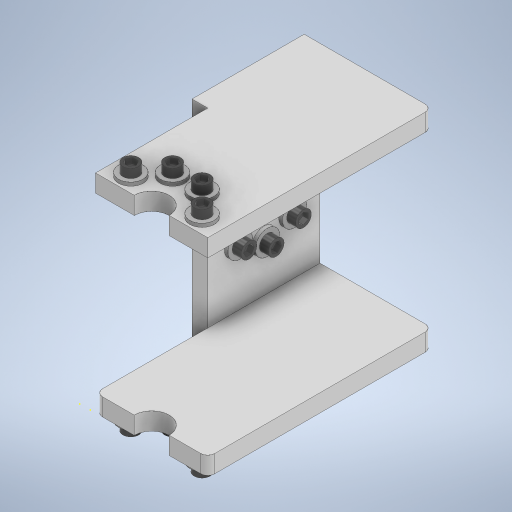
# Autodesk Inventor part: link_manip
Saved by Autodesk Inventor 2024 (Build 280153000, 153)
## iProperties
Created: 2024-10-14
Part Number: link_manip
Material: Genérico
Document SubType Name: Modeling
Designer: robof
Density: 1 g/cm^3
Appearance: Padrão
Author: robof
Autodesk Inventor part; units mm, degrees
ref_plane "YZ Plane" through (0, 0, 0) normal (1, 0, 0) x (0, 1, 0)
ref_plane "XZ Plane" through (0, 0, 0) normal (0, 1, 0) x (-1, 0, 0)
ref_plane "XY Plane" through (0, 0, 0) normal (0, 0, 1) x (1, 0, 0)
sketch "Esboço1" plane through (0, 0, 0) normal (0, 1, 0) x (-1, 0, 0)
  line L0 (0, 0) -> (-32, 0)
  line L1 (-32, 0) -> (-32, -64)
  line L2 (-32, -64) -> (0, -64)
  line L3 (0, -64) -> (0, 0)
  dimension "d0" = 32
  dimension "d1" = 64
  constraints: 8 end point, 2 parallel, 1 horizontal, 1 perpendicular
  measures "d0" distance of L2.end L1.end
  measures "d1" distance of L1.end L0.end
extrude "Extrusão1" add sketch "Esboço1" along normal blind 5
sketch "Esboço2" plane through (0, 5, 0) normal (0, 1, 0) x (1, 0, 0)
  line L0 (32, 64) -> (0, 64) projected
  line L1 (0, 64) -> (-4.5, 64)
  line L2 (-4.5, 64) -> (-4.5, 35.5)
  line L3 (-4.5, 35.5) -> (0, 35.5)
  line L4 (0, 35.5) -> (0, 64)
  point P0 (0, 0)
  dimension "d4" = 4.5
  dimension "d5" = 28.5
  constraints: 8 end point, 2 parallel, 1 horizontal, 1 perpendicular
  measures "d4" distance of L3.end L2.end
  measures "d5" distance of L2.end L1.end
extrude "Extrusão2" add sketch "Esboço2" along normal blind 59.3
sketch "Esboço3" plane through (0, 5, 0) normal (0, -1, 0) x (1, 0, 0)
  line L0 (0, -64) -> (-4.5, -64) projected
  line L1 (0, -64) -> (0, -35.5) projected
  line L2 (-4.5, -64) -> (0, -64)
  line L3 (0, -64) -> (0, -35.5)
  line L4 (0, -35.5) -> (-4.5, -35.5)
  line L5 (-4.5, -35.5) -> (-4.5, -64)
  point P0 (0, 0)
  constraints: 8 end point, 2 parallel, 1 horizontal, 1 perpendicular
extrude "Extrusão3" add sketch "Esboço3" along normal blind 5
sketch "Esboço4" plane through (0, 64.3, 0) normal (0, 1, 0) x (1, 0, 0)
  line L0 (-4.5, 35.5) -> (-4.5, 64) projected
  line L1 (0, 35.5) -> (0, 64) projected
  line L2 (-4.5, 64) -> (0, 64)
  line L3 (0, 64) -> (0, 35.5)
  line L4 (0, 35.5) -> (-4.5, 35.5)
  line L5 (-4.5, 35.5) -> (-4.5, 64)
  point P0 (0, 0)
  constraints: 8 end point, 2 parallel, 1 horizontal, 1 perpendicular
extrude "Extrusão4" cut sketch "Esboço4" against normal blind 5
sketch "Esboço5" plane through (0, 59.3, 0) normal (0, 1, 0) x (1, 0, 0)
  line L0 (0, 64) -> (0, 35.5) projected
  line L1 (0, 0) -> (32, 0) projected
  line L2 (0, 64) -> (32, 64)
  line L3 (32, 64) -> (32, 0)
  line L4 (32, 0) -> (0, 0)
  line L5 (0, 0) -> (0, 64)
  constraints: 8 end point, 2 parallel, 1 horizontal, 1 perpendicular
extrude "Extrusão5" add sketch "Esboço5" against normal blind 5
sketch "Esboço6" plane through (0, 59.3, 0) normal (0, 1, 0) x (1, 0, 0)
  line L0 (0, 0) -> (32, 0) projected
  circle A0 centre (16, 0) radius 4.975
  point P0 (20.975, 0)
  point P1 (11.025, 0)
  dimension "d14" = 9.95
  constraints: 1 centre point, 1 midpoint
  measures "d14" diameter of A0
extrude "Extrusão6" cut sketch "Esboço6" against normal blind 100 contours A0 L0 picked at (17.4684, 0.7707)
sketch "Esboço7" plane through (0, 0, 0) normal (0, -1, 0) x (1, 0, 0)
  arc A0 (11.025, 0) -> (20.975, 0) centre (16, 0) ccw projected
  line L0 (16, 0) -> (16, -11.7992)
  line L1 (16, 0) -> (24.7548, -8.7548)
  line L2 (16, 0) -> (28.3812, 0) construction
  line L3 (16, 0) -> (21.1285, -12.3812)
  line L4 (16, 0) -> (29.4013, 0) construction
  line L5 (16, 0) -> (27.5056, -4.7658)
  line L6 (16, 0) -> (28.4535, 0) construction
  arc A1 (11.025, 0) -> (20.975, 0) centre (16, 0) ccw
  line L7 (16, 0) -> (7.2452, -8.7548)
  line L8 (16, 0) -> (10.8715, -12.3812)
  line L9 (16, 0) -> (4.4944, -4.7658)
  line L10 (16, 0) -> (26.1627, -4.2095)
  circle A2 centre (26.1627, -4.2095) radius 3.5
  circle A3 centre (20.2095, -10.1627) radius 3.5
  circle A4 centre (5.8373, -4.2095) radius 3.5
  circle A5 centre (11.7905, -10.1627) radius 3.5
  point P0 (0, 0)
  dimension "d17" = 45
  dimension "d18" = 67.5
  dimension "d19" = 22.5
  dimension "d20" = 11
  dimension "d21" = 7
  constraints: 22 end point, 8 symmetric about line, 5 centre point, 3 equal length, 3 horizontal, 2 point on circle, 1 coincident, 1 point on line, 1 vertical, 4 other
  measures "d17" angle of L1 L2
  measures "d18" angle of L3 L4
  measures "d19" angle of L5 L6
  measures "d20" distance of L0.start L10.end
  measures "d21" diameter of A2
extrude "Extrusão7" add sketch "Esboço7" along normal blind 1 contours A2 | A3 | A5 | A4
sketch "Esboço8" plane through (5.8373, -1, -4.2095) normal (0, -1, 0) x (1, 0, 0)
  circle A0 centre (0, 0) radius 2.25
  circle A1 centre (5.9532, -5.9532) radius 3.5 projected
  circle A2 centre (5.9532, -5.9532) radius 2.25
  circle A3 centre (14.3722, -5.9532) radius 3.5 projected
  circle A4 centre (14.3722, -5.9532) radius 2.25
  circle A5 centre (20.3253, 0) radius 3.5 projected
  circle A6 centre (20.3253, 0) radius 2.25
  point P0 (-5.8373, 4.2095)
  dimension "d24" = 4.5
  dimension "d25" = 4.5
  dimension "d26" = 4.5
  dimension "d27" = 4.5
  constraints: 4 centre point, 3 coincident
  measures "d24" diameter of A0
  measures "d25" diameter of A2
  measures "d26" diameter of A4
  measures "d27" diameter of A6
extrude "Extrusão8" add sketch "Esboço8" along normal blind 2.5 contours A0 | A2 | A4 | A6
sketch "Esboço9" plane through (5.8373, -3.5, -4.2095) normal (0, -1, 0) x (1, 0, 0)
  line L0 (-1.5951, 0) -> (-0.7976, 1.3814)
  line L1 (-0.7976, 1.3814) -> (0.7976, 1.3814)
  line L2 (0.7976, 1.3814) -> (1.5951, 0)
  line L3 (1.5951, 0) -> (0.7976, -1.3814)
  line L4 (0.7976, -1.3814) -> (-0.7976, -1.3814)
  line L5 (-0.7976, -1.3814) -> (-1.5951, 0)
  arc A0 (5.1877, 4.2095) -> (15.1377, 4.2095) centre (10.1627, 4.2095) ccw projected
  line L6 (10.1627, 4.2095) -> (-1.1963, -7.1495)
  line L7 (10.1627, 4.2095) -> (26.2267, 4.2095) construction
  line L8 (10.1627, 4.2095) -> (19.9498, -5.5776)
  line L9 (10.1627, 4.2095) -> (10.1627, -8.2153)
  line L10 (5.9532, -7.5483) -> (7.3346, -6.7507)
  line L11 (7.3346, -6.7507) -> (7.3346, -5.1556)
  line L12 (7.3346, -5.1556) -> (5.9532, -4.3581)
  line L13 (5.9532, -4.3581) -> (4.5718, -5.1556)
  line L14 (4.5718, -5.1556) -> (4.5718, -6.7507)
  line L15 (4.5718, -6.7507) -> (5.9532, -7.5483)
  line L16 (21.9205, 0) -> (21.1229, 1.3814)
  line L17 (21.1229, 1.3814) -> (19.5278, 1.3814)
  line L18 (19.5278, 1.3814) -> (18.7302, 0)
  line L19 (18.7302, 0) -> (19.5278, -1.3814)
  line L20 (19.5278, -1.3814) -> (21.1229, -1.3814)
  line L21 (21.1229, -1.3814) -> (21.9205, 0)
  line L22 (14.3722, -7.5483) -> (12.9908, -6.7507)
  line L23 (12.9908, -6.7507) -> (12.9908, -5.1556)
  line L24 (12.9908, -5.1556) -> (14.3722, -4.3581)
  line L25 (14.3722, -4.3581) -> (15.7536, -5.1556)
  line L26 (15.7536, -5.1556) -> (15.7536, -6.7507)
  line L27 (15.7536, -6.7507) -> (14.3722, -7.5483)
  point P0 (-5.8373, 4.2095)
  point P1 (0, 0)
  point P2 (5.9532, -5.9532)
  point P3 (20.3253, 0)
  point P4 (21.5217, -7.1495)
  point P5 (14.3722, -5.9532)
  dimension "d30" = 135
  constraints: 56 end point, 22 symmetric about line, 1 equal length, 1 horizontal, 1 vertical, 13 other
  measures "d30" angle of L6 L7
extrude "Extrusão9" cut sketch "Esboço9" against normal blind 1.5 contours L0 L1 L2 L3 L4 L5 | L15 L14 L13 L12 L11 L10 | L21 L20 L19 L18 L17 L16 | L22 L23 L24 L25 L26 L27
sketch "Esboço10" plane through (0, 59.3, 0) normal (0, 1, 0) x (1, 0, 0)
  circle A0 centre (20.2095, 10.1627) radius 3.5 projected
  circle A1 centre (20.2095, 10.1627) radius 3.5
  circle A2 centre (26.1627, 4.2095) radius 2.25 projected
  circle A3 centre (26.1627, 4.2095) radius 3.5
  circle A4 centre (11.7905, 10.1627) radius 2.25 projected
  circle A5 centre (11.7905, 10.1627) radius 3.5
  circle A6 centre (5.8373, 4.2095) radius 3.5
  point P0 (0, 0)
  constraints: 4 centre point, 3 coincident
extrude "Extrusão10" add sketch "Esboço10" along normal blind 1 contours A0 | A2 | A3 | A4 | A5 | A6
sketch "Esboço11" plane through (5.8373, 60.3, -4.2095) normal (0, 1, 0) x (1, 0, 0)
  circle A0 centre (0, 0) radius 2.25
  circle A1 centre (5.9532, 5.9532) radius 2.25 projected
  circle A2 centre (5.9532, 5.9532) radius 2.25
  circle A3 centre (14.3722, 5.9532) radius 3.5 projected
  circle A4 centre (14.3722, 5.9532) radius 2.25
  circle A5 centre (20.3253, 0) radius 3.5 projected
  circle A6 centre (20.3253, 0) radius 2.25
  point P0 (-5.8373, -4.2095)
  constraints: 4 centre point, 3 coincident
extrude "Extrusão11" add sketch "Esboço11" along normal blind 2.5 contours A0 | A1 | A4 | A6
sketch "Esboço12" plane through (5.8373, 62.8, -4.2095) normal (0, 1, 0) x (1, 0, 0)
  circle A0 centre (0, 0) radius 2.25 projected
  line L0 (0.7976, 1.3814) -> (-0.7976, 1.3814) projected
  line L1 (0.7976, 1.3814) -> (1.5951, 0)
  line L2 (1.5951, 0) -> (0.7976, -1.3814)
  line L3 (0.7976, -1.3814) -> (-0.7976, -1.3814)
  line L4 (-0.7976, -1.3814) -> (-1.5951, 0)
  line L5 (-1.5951, 0) -> (-0.7976, 1.3814)
  line L6 (-0.7976, 1.3814) -> (0.7976, 1.3814)
  circle A1 centre (5.9532, 5.9532) radius 2.25 projected
  line L7 (7.3346, 6.7507) -> (5.9532, 7.5483) projected
  line L8 (5.9532, 7.5483) -> (7.3346, 6.7507)
  line L9 (7.3346, 6.7507) -> (7.3346, 5.1556)
  line L10 (7.3346, 5.1556) -> (5.9532, 4.3581)
  line L11 (5.9532, 4.3581) -> (4.5718, 5.1556)
  line L12 (4.5718, 5.1556) -> (4.5718, 6.7507)
  line L13 (4.5718, 6.7507) -> (5.9532, 7.5483)
  circle A2 centre (14.3722, 5.9532) radius 2.25 projected
  line L14 (12.9908, 5.1556) -> (14.3722, 4.3581) projected
  line L15 (12.9908, 5.1556) -> (12.9908, 6.7507)
  line L16 (12.9908, 6.7507) -> (14.3722, 7.5483)
  line L17 (14.3722, 7.5483) -> (15.7536, 6.7507)
  line L18 (15.7536, 6.7507) -> (15.7536, 5.1556)
  line L19 (15.7536, 5.1556) -> (14.3722, 4.3581)
  line L20 (14.3722, 4.3581) -> (12.9908, 5.1556)
  circle A3 centre (20.3253, 0) radius 2.25 projected
  line L21 (19.5277, -1.3814) -> (18.7302, 0.0001)
  line L22 (18.7302, 0.0001) -> (19.5278, 1.3815)
  line L23 (19.5278, 1.3815) -> (21.123, 1.3814)
  line L24 (21.123, 1.3814) -> (21.9205, -0.0001)
  line L25 (21.9205, -0.0001) -> (21.1229, -1.3815)
  line L26 (21.1229, -1.3815) -> (19.5277, -1.3814)
  point P0 (-5.8373, -4.2095)
  constraints: 48 end point, 4 coincident, 1 point on line, 52 other
extrude "Extrusão12" cut sketch "Esboço12" against normal blind 1.5 contours L1 L2 L3 L4 L5 L0 | L9 L10 L11 L12 L13 L7 | L15 L16 L17 L18 L19 L14 | L21 L22 L23 L24 L25 L26
fillet "Arredondamento1" radius 2 6 edges at (0, 2.5, 0) (32, 2.5, 0) (32, 2.5, -64) (32, 56.8, -64) (0, 56.8, -35.5) (0, 2.5, -35.5)
sketch "Esboço13" plane through (0, 5, -35.5) normal (1, 0, 0) x (0, 0, -1)
  line L0 (0, 0) -> (0, 49.3) projected
  line L1 (0, 24.65) -> (28.5, 24.65)
  line L2 (28.5, 0) -> (28.5, 49.3) projected
  circle A0 centre (14.25, 24.65) radius 5.85
  point P0 (-35.5, -5)
  dimension "d40" = 11.7
  constraints: 3 midpoint, 2 end point, 1 centre point
  measures "d40" diameter of A0
extrude "Extrusão13" cut sketch "Esboço13" against normal blind 1.5
sketch "Esboço14" plane through (-1.5, 29.65, -49.75) normal (1, 0, 0) x (0, 0, -1)
  point P0 (-49.75, -29.65)
sketch "Esboço15" plane through (0, 5, -35.5) normal (1, 0, 0) x (0, 0, -1)
  circle A0 centre (14.25, 24.65) radius 5.85 projected
  circle A1 centre (14.25, 24.65) radius 5.85
  point P0 (-35.5, -5)
  constraints: 1 centre point, 1 coincident
extrude "Extrusão14" add sketch "Esboço15" against normal blind 10
sketch "Esboço16" plane through (0, 5, -35.5) normal (1, 0, 0) x (0, 0, -1)
  line L0 (0, 0) -> (0, 49.3) projected
  line L1 (0, 24.65) -> (28.5, 24.65)
  line L2 (28.5, 0) -> (28.5, 49.3) projected
  circle A0 centre (14.25, 24.65) radius 5.85
  point P0 (-35.5, -5)
  constraints: 3 midpoint, 2 end point, 1 centre point
extrude "Extrusão15" cut sketch "Esboço16" against normal blind 10
sketch "Esboço17" plane through (0, 5, -35.5) normal (1, 0, 0) x (0, 0, -1)
  line L0 (14.25, 24.65) -> (28.5632, 24.65) construction
  line L1 (0, 0) -> (0, 49.3) projected
  line L2 (0, 24.65) -> (28.5632, 24.65)
  circle A0 centre (14.25, 24.65) radius 5.85 projected
  circle A1 centre (14.25, 24.65) radius 5.85
  point P0 (-35.5, -5)
  constraints: 4 end point, 1 centre point, 1 coincident, 1 collinear, 1 horizontal, 1 midpoint
extrude "Extrusão16" add sketch "Esboço17" against normal blind 5
sketch "Esboço18" plane through (-4.5, 0, -35.5) normal (0, 0, 1) x (1, 0, 0)
  line L0 (0, 59.3) -> (4.5, 59.3)
  line L1 (4.5, 59.3) -> (4.5, 0)
  line L2 (4.5, 0) -> (0, 0)
  line L3 (0, 0) -> (0, 59.3)
  constraints: 8 end point, 2 parallel, 1 horizontal, 1 perpendicular
extrude "Extrusão17" add sketch "Esboço18" along normal blind 3.5
sketch "Esboço19" plane through (-5, 29.65, -49.75) normal (-1, 0, 0) x (0, 0, 1)
  circle A0 centre (0, 0) radius 5.85 projected
  circle A1 centre (0, 0) radius 5.85
  point P0 (49.75, -29.65)
  constraints: 1 centre point, 1 coincident
extrude "Extrusão18" cut sketch "Esboço19" against normal blind 0.5
sketch "Esboço20" plane through (0, 5, -64) normal (1, 0, 0) x (0, 0, -1)
  line L0 (-32, 54.3) -> (-32, -5) projected
  line L1 (-32, 24.65) -> (0, 24.65)
  line L2 (0, -5) -> (0, 54.3) projected
  circle A0 centre (-16, 24.65) radius 5.9
  line L3 (-16, 24.65) -> (-8.2218, 16.8718)
  line L4 (-16, 24.65) -> (-5, 24.65) construction
  line L5 (-16, 24.65) -> (-16, 13.65)
  line L6 (-16, 24.65) -> (-8.2218, 32.4282)
  line L7 (-16, 24.65) -> (-16, 35.65)
  line L8 (-16, 24.65) -> (-23.7782, 16.8718)
  line L9 (-16, 24.65) -> (-23.7782, 32.4282)
  circle A1 centre (-8.2218, 32.4282) radius 3.5
  circle A2 centre (-16, 35.65) radius 3.5
  circle A3 centre (-23.7782, 32.4282) radius 3.5
  circle A4 centre (-23.7782, 16.8718) radius 3.5
  circle A5 centre (-16, 13.65) radius 3.5
  circle A6 centre (-8.2218, 16.8718) radius 3.5
  line L10 (-16, 24.65) -> (-5, 24.65)
  circle A7 centre (-5, 24.65) radius 3.5
  line L11 (-16, 24.65) -> (-27, 24.65)
  circle A8 centre (-27, 24.65) radius 3.5
  point P0 (-64, -5)
  point P1 (-30.5, 24.65)
  point P2 (-23.5, 24.65)
  dimension "d60" = 11.8
  dimension "d61" = 11
  dimension "d62" = 45
  dimension "d63" = 11
  dimension "d64" = 7
  dimension "d65" = 7
  dimension "d66" = 7
  dimension "d67" = 7
  dimension "d68" = 7
  dimension "d69" = 7
  dimension "d70" = 11
  dimension "d71" = 7
  dimension "d72" = 11
  dimension "d73" = 7
  constraints: 20 end point, 9 centre point, 8 coincident, 4 symmetric about line, 3 midpoint, 1 collinear, 1 equal length, 1 horizontal, 1 point on line, 1 vertical
  measures "d60" diameter of A0
  measures "d61" distance of L3.start L3.end
  measures "d62" angle of L3 L4
  measures "d63" distance of L3.start L5.end
  measures "d64" diameter of A1
  measures "d65" diameter of A2
  measures "d66" diameter of A3
  measures "d67" diameter of A4
  measures "d68" diameter of A5
  measures "d69" diameter of A6
  measures "d70" distance of L3.start L4.end
  measures "d71" diameter of A7
  measures "d72" distance of L3.start L11.end
  measures "d73" diameter of A8
extrude "Extrusão19" add sketch "Esboço20" along normal blind 1 contours L1 A8 | A3 | A2 | A1 | A7 L1 | L1 A7 | A6 | A5 | A4 | A0 L9 L1 | L1 L8 A0 | L6 A0 L1 | L1 A0 L3 | L3 A0 L5 | L7 A0 L6 | L9 A0 L7 | L5 A0 L8 picked at (-24.7006, 24.3708)
sketch "Esboço21" plane through (0, 5, -64) normal (1, 0, 0) x (0, 0, -1)
  line L0 (-23.5, 24.65) -> (-30.5, 24.65) projected
  circle A0 centre (-27, 24.65) radius 3.5
  point P0 (-64, -5)
  constraints: 1 midpoint, 3 other
extrude "Extrusão20" add sketch "Esboço21" along normal blind 1 contours L0 A0 picked at (-26.1267, 25.4236)
sketch "Esboço22" plane through (1, 29.65, -48) normal (1, 0, 0) x (0, 0, -1)
  circle A0 centre (0, 0) radius 5.9 projected
  circle A1 centre (0, 0) radius 5.9
  point P0 (-48, -29.65)
  constraints: 1 centre point, 1 coincident
extrude "Extrusão21" cut sketch "Esboço22" against normal blind 3
sketch "Esboço23" plane through (-2, 29.65, -48) normal (1, 0, 0) x (0, 0, -1)
  circle A0 centre (0, 0) radius 5.9 projected
  circle A1 centre (0, 0) radius 5.9
  point P0 (-48, -29.65)
  constraints: 1 centre point, 1 coincident
extrude "Extrusão22" cut sketch "Esboço23" against normal blind 20
sketch "Esboço24" plane through (1, 29.65, -59) normal (1, 0, 0) x (0, 0, -1)
  circle A0 centre (0, 0) radius 3.5 projected
  circle A1 centre (0, 0) radius 2.25
  circle A2 centre (-11, 0) radius 5.9 projected
  line L0 (-11, 0) -> (2.7014, 0) construction
  circle A3 centre (-11, -11) radius 2.25
  line L1 (-11, 0) -> (4.8079, 0)
  circle A4 centre (-11, -11) radius 2.25
  circle A5 centre (0, 0) radius 2.25
  circle A6 centre (-22, 0) radius 2.25
  circle A7 centre (-11, 11) radius 3.5 projected
  circle A8 centre (-11, 11) radius 2.25
  circle A9 centre (-3.2218, 7.7782) radius 2.25
  circle A10 centre (-11, 11) radius 2.25
  circle A11 centre (-18.7782, 7.7782) radius 2.25
  circle A12 centre (-22, 0) radius 2.25
  circle A13 centre (-18.7782, -7.7782) radius 2.25
  circle A14 centre (-11, -11) radius 2.25
  circle A15 centre (-3.2218, -7.7782) radius 2.25
  point P0 (-59, -29.65)
  dimension "d82" = 4.5
  dimension "d84" = 4.5
  dimension "d87" = 360
  constraints: 13 centre point, 4 end point, 2 coincident, 1 horizontal, 17 other
  measures "d82" diameter of A1
  measures "d84" diameter of A8
extrude "Extrusão23" add sketch "Esboço24" along normal blind 2.5 contours L1 A1 | A1 L1 | A3 | A6 | A8 | A9 | A11 | A13 | A15
sketch "Esboço25" plane through (3.5, 37.4282, -55.7782) normal (1, 0, 0) x (0, 0, -1)
  circle A0 centre (0, 0) radius 2.25 projected
  line L0 (-1.5521, 0) -> (-0.7761, 1.3442)
  line L1 (-0.7761, 1.3442) -> (0.7761, 1.3442)
  line L2 (0.7761, 1.3442) -> (1.5521, 0)
  line L3 (1.5521, 0) -> (0.7761, -1.3442)
  line L4 (0.7761, -1.3442) -> (-0.7761, -1.3442)
  line L5 (-0.7761, -1.3442) -> (-1.5521, 0)
  circle A1 centre (-7.7782, -7.7782) radius 5.9 projected
  circle A2 centre (-7.7782, -7.7782) radius 5.9
  line L6 (-6.6806, 4.3194) -> (-6.2789, 2.8201)
  line L7 (-8.1799, 4.7211) -> (-6.6806, 4.3194)
  line L8 (-9.2774, 3.6235) -> (-8.1799, 4.7211)
  line L9 (-8.8757, 2.1243) -> (-9.2774, 3.6235)
  line L10 (-6.2789, 2.8201) -> (-7.3765, 1.7226)
  line L11 (-7.3765, 1.7226) -> (-8.8757, 2.1243)
  line L12 (-15.5563, 1.5521) -> (-14.2122, 0.7761)
  line L13 (-16.9005, 0.7761) -> (-15.5563, 1.5521)
  line L14 (-16.9005, -0.7761) -> (-16.9005, 0.7761)
  line L15 (-15.5563, -1.5521) -> (-16.9005, -0.7761)
  line L16 (-14.2122, 0.7761) -> (-14.2122, -0.7761)
  line L17 (-14.2122, -0.7761) -> (-15.5563, -1.5521)
  line L18 (-19.8757, -6.6806) -> (-18.3765, -6.2789)
  line L19 (-20.2774, -8.1799) -> (-19.8757, -6.6806)
  line L20 (-19.1799, -9.2774) -> (-20.2774, -8.1799)
  line L21 (-17.6806, -8.8757) -> (-19.1799, -9.2774)
  line L22 (-18.3765, -6.2789) -> (-17.2789, -7.3765)
  line L23 (-17.2789, -7.3765) -> (-17.6806, -8.8757)
  line L24 (-17.1085, -15.5563) -> (-16.3324, -14.2122)
  line L25 (-16.3324, -16.9005) -> (-17.1085, -15.5563)
  line L26 (-14.7803, -16.9005) -> (-16.3324, -16.9005)
  line L27 (-14.0042, -15.5563) -> (-14.7803, -16.9005)
  line L28 (-16.3324, -14.2122) -> (-14.7803, -14.2122)
  line L29 (-14.7803, -14.2122) -> (-14.0042, -15.5563)
  line L30 (-8.8757, -19.8757) -> (-9.2774, -18.3765)
  line L31 (-7.3765, -20.2774) -> (-8.8757, -19.8757)
  line L32 (-6.2789, -19.1799) -> (-7.3765, -20.2774)
  line L33 (-6.6806, -17.6806) -> (-6.2789, -19.1799)
  line L34 (-9.2774, -18.3765) -> (-8.1799, -17.2789)
  line L35 (-8.1799, -17.2789) -> (-6.6806, -17.6806)
  line L36 (0, -17.1085) -> (-1.3442, -16.3324)
  line L37 (1.3442, -16.3324) -> (0, -17.1085)
  line L38 (1.3442, -14.7803) -> (1.3442, -16.3324)
  line L39 (0, -14.0042) -> (1.3442, -14.7803)
  line L40 (-1.3442, -16.3324) -> (-1.3442, -14.7803)
  line L41 (-1.3442, -14.7803) -> (0, -14.0042)
  line L42 (4.3194, -8.8757) -> (2.8201, -9.2774)
  line L43 (4.7211, -7.3765) -> (4.3194, -8.8757)
  line L44 (3.6235, -6.2789) -> (4.7211, -7.3765)
  line L45 (2.1243, -6.6806) -> (3.6235, -6.2789)
  line L46 (2.8201, -9.2774) -> (1.7226, -8.1799)
  line L47 (1.7226, -8.1799) -> (2.1243, -6.6806)
  point P0 (-55.7782, -37.4282)
  dimension "d93" = 360
  constraints: 96 end point, 2 coincident, 1 centre point, 110 other
extrude "Extrusão24" cut sketch "Esboço25" against normal blind 1.5 contours L0 L1 L2 L3 L4 L5 | L6 L10 L11 L9 L8 L7 | L12 L16 L17 L15 L14 L13 | L18 L22 L23 L21 L20 L19 | L24 L28 L29 L27 L26 L25 | L30 L34 L35 L33 L32 L31 | L36 L40 L41 L39 L38 L37 | L42 L46 L47 L45 L44 L43
sketch "Esboço26" plane through (-4.5, 0, -64) normal (-1, 0, 0) x (0, 0, 1)
  point P0 (64, 0)
